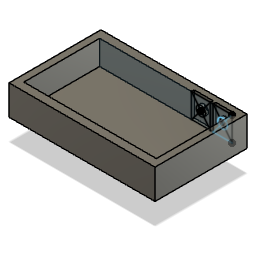
VCR (Autodesk Fusion 360 design; units mm, degrees)
Autodesk Fusion 360 part; units mm, degrees
note: some values were not read from the file. Set by a fixed rule: which sketch regions a step uses.
sketch "Sketch1" plane through (0, 0, 0) normal (0, 1, 0) x (1, 0, 0)
  line L0 (27, 17) -> (-27, 17)
  line L1 (-27, 17) -> (-27, -17)
  line L2 (-27, -17) -> (27, -17)
  line L3 (27, -17) -> (27, 17)
  line L4 (27, 17) -> (-27, -17) construction
  line L5 (-27, 17) -> (27, -17) construction
  dimension "d1" = 54
  dimension "d2" = 34
  constraint horizontal L0
  constraint perpendicular L0 L1
  constraint parallel L0 L2
  constraint parallel L1 L3
  constraint coincident L4 origin
  constraint coincident L5 origin
  measures "d1" distance of L1.end L2.end
  measures "d2" distance of L0.end L1.end
extrude "Extrude1" add sketch "Sketch1" along normal blind 11
sketch "Sketch2" plane through (0, 11, 0) normal (0, 1, 0) x (-1, 0, 0)
  line L0 (-27, 17) -> (-27, -17)
  line L1 (-27, -17) -> (27, -17)
  line L2 (27, -17) -> (27, 17)
  line L3 (27, 17) -> (-27, 17)
  line L4 (-24.5, -14) -> (24.5, -14)
  line L5 (24.5, -14) -> (24.5, 14)
  line L6 (24.5, 14) -> (-24.5, 14)
  line L7 (-24.5, 14) -> (-24.5, -14)
  line L8 (-24.5, -14) -> (24.5, 14) construction
  line L9 (24.5, -14) -> (-24.5, 14) construction
  dimension "d5" = 49
  dimension "d6" = 28
  constraint horizontal L4
  constraint perpendicular L4 L5
  constraint parallel L4 L6
  constraint parallel L5 L7
  constraint coincident L8 origin
  constraint coincident L9 origin
  measures "d5" distance of L5.end L6.end
  measures "d6" distance of L4.end L5.end
extrude "Extrude2" cut sketch "Sketch2" against normal blind 9 contours L4 L5 L6 L7
sketch "Sketch4" plane through (0, 0, -14) normal (0, 0, 1) x (1, 0, 0)
  line L0 (24.5, 11) -> (-24.5, 11)
  line L1 (-24.5, 11) -> (-24.5, 2)
  line L2 (-24.5, 2) -> (24.5, 2)
  line L3 (24.5, 2) -> (24.5, 11)
  line L4 (24.5, 11) -> (17.5, 11)
  line L5 (17.5, 11) -> (17.5, 2)
  line L6 (17.5, 2) -> (24.5, 2)
  line L7 (24.5, 2) -> (24.5, 11)
  line L8 (24.5, 2) -> (17.5, 11)
  line L9 (17.5, 2) -> (24.5, 11)
  circle A0 centre (21, 6.5) radius 1.75
  line L10 (17.5, 11) -> (16.5, 11)
  line L11 (16.5, 11) -> (16.5, 2)
  line L12 (16.5, 2) -> (17.5, 2)
  line L13 (17.5, 2) -> (17.5, 11)
  line L14 (16.5, 11) -> (9.5, 11)
  line L15 (9.5, 11) -> (9.5, 2)
  line L16 (9.5, 2) -> (16.5, 2)
  line L17 (16.5, 2) -> (16.5, 11)
  line L18 (9.5, 11) -> (16.5, 2)
  line L19 (9.5, 2) -> (16.5, 11)
  circle A1 centre (13, 6.5) radius 1.75
  dimension "d9" = 7
  dimension "d10" = 3.5
  dimension "d13" = 1
  dimension "d14" = 9
  dimension "d15" = 7
  dimension "d16" = 9
  dimension "d17" = 3.5
  constraint horizontal L4
  constraint vertical L5
  constraint horizontal L6
  constraint vertical L7
  constraint coincident L0.start L3.end
  constraint coincident L2.end L3.start
  constraint midpoint L9 A0.centre
  constraint horizontal L10
  constraint vertical L11
  constraint horizontal L12
  constraint vertical L13
  constraint horizontal L14
  constraint vertical L15
  constraint horizontal L16
  constraint vertical L17
  constraint midpoint L19 A1.centre
  measures "d9" distance of L0.start L4.end
  measures "d10" diameter of A0
  measures "d13" distance of L4.end L10.end
  measures "d14" distance of L4.end L5.end
  measures "d15" distance of L10.end L14.end
  measures "d16" distance of L10.end L11.end
  measures "d17" diameter of A1
extrude "Extrude5" cut sketch "Sketch4" against normal blind 1 contours L0 L4 L8 L9 A0 | L3 L7 L8 L9 A0 | L5 L8 L9 A0 L13 | L2 L6 L8 L9 A0 | L0 L14 L18 L19 A1 | L11 L17 L18 L19 A1 | L15 L18 L19 A1 | L2 L16 L18 L19 A1
extrude "Extrude3" cut sketch "Sketch4" against normal blind 3 contours L8 L9 A0 | L8 L9 A0 | L8 L9 A0 | L8 L9 A0 | L18 L19 A1 | L18 L19 A1 | L18 L19 A1 | L18 L19 A1
sketch "Sketch5" plane through (0, 0, -17) normal (0, 0, -1) x (-1, 0, 0)
  circle A0 centre (-21, 6.5) radius 1.75
  circle A1 centre (-13, 6.5) radius 1.75
  line L0 (-27, 0) -> (27, 0)
  line L1 (27, 0) -> (27, 11)
  line L2 (27, 11) -> (-27, 11)
  line L3 (-27, 11) -> (-27, 0)
  line L4 (23, 4) -> (-4, 4)
  line L5 (-4, 4) -> (-4, 9)
  line L6 (-4, 9) -> (23, 9)
  line L7 (23, 9) -> (23, 4)
  dimension "d20" = 5
  dimension "d21" = 27
  constraint horizontal L4
  constraint vertical L5
  constraint horizontal L6
  constraint vertical L7
  measures "d20" distance of L4.start L6.end
  measures "d21" distance of L5.end L6.end
extrude "Extrude4" cut sketch "Sketch5" against normal blind 1 contours L4 L5 L6 L7
sketch "Sketch6" plane through (0, 0, 0) normal (0, -1, 0) x (1, 0, 0)
  line L0 (27, -17) -> (27, 17)
  line L1 (27, 17) -> (-27, 17)
  line L2 (-27, 17) -> (-27, -17)
  line L3 (-27, -17) -> (27, -17)
  circle A0 centre (0, 0) radius 10.5
  dimension "d24" = 21
  constraint coincident A0.centre origin
  measures "d24" diameter of A0
extrude "Extrude6" add sketch "Sketch6" along normal blind 8 contours A0
fillet "Fillet1" radius 10.5 1 faces at (-2.9623, -8, 1.0316)
sketch "Sketch7" plane through (0, -8, 0) normal (0, -1, 0) x (1, 0, 0)
  circle A0 centre (0, 0) radius 0.302
  line L0 (10.5, 1.5) -> (-10.5, 1.5)
  line L1 (-10.5, 1.5) -> (-10.5, -1.5)
  line L2 (-10.5, -1.5) -> (10.5, -1.5)
  line L3 (10.5, -1.5) -> (10.5, 1.5)
  line L4 (10.5, 1.5) -> (-10.5, -1.5) construction
  line L5 (-10.5, 1.5) -> (10.5, -1.5) construction
  dimension "d29" = 21
  dimension "d30" = 3
  constraint horizontal L0
  constraint perpendicular L0 L1
  constraint parallel L0 L2
  constraint parallel L1 L3
  constraint coincident L4 A0.centre
  constraint coincident L5 A0.centre
  constraint coincident A0.centre origin
  measures "d29" distance of L1.end L2.end
  measures "d30" distance of L0.end L1.end
extrude "Extrude7" cut sketch "Sketch7" against normal blind 6 contours A0 | L0 L1 L2 L3
sketch "Sketch8" plane through (0, -2, 0) normal (0, -1, 0) x (1, 0, 0)
  arc A0 (-9.6732, 1.5) -> (-9.6732, -1.5) centre (0, 0) ccw
  line L0 (-9.6732, -1.5) -> (9.6732, -1.5)
  arc A1 (9.6732, -1.5) -> (9.6732, 1.5) centre (0, 0) ccw
  line L1 (9.6732, 1.5) -> (-9.6732, 1.5)
  circle A2 centre (-5.5, 0) radius 1
  circle A3 centre (6.5, 0) radius 1
  dimension "d33" = 2
  dimension "d34" = 2
  measures "d33" diameter of A2
  measures "d34" diameter of A3
extrude "Extrude8" cut sketch "Sketch8" against normal blind 2 contours A2 | A3
